Light Switch Plate_v1 (Autodesk Fusion 360 design; units mm, degrees)
Autodesk Fusion 360 part; units mm, degrees
note: some values were not read from the file. Set by a fixed rule: which sketch regions a step uses.
sketch "Sketch1" plane through (0, 0, 0) normal (0, 0, 1) x (1, 0, 0)
  line L0 (-35, 57) -> (35, 57)
  line L1 (35, 57) -> (35, -57)
  line L2 (35, -57) -> (-35, -57)
  line L3 (-35, -57) -> (-35, 57)
  line L4 (-50, 0) -> (50, 0)
  circle A0 centre (0.0006, 30.16) radius 3.5
  circle A1 centre (0.0006, -30.16) radius 3.5
  line L5 (0, 65) -> (0, -65)
  line L6 (5.155, 0) -> (5.155, 11.965)
  line L7 (5.155, 11.965) -> (0, 11.965)
  line L8 (-5.155, 11.965) -> (0, 11.965)
  line L9 (-5.155, 0) -> (-5.155, 11.965)
  line L10 (-5.155, 0) -> (-5.155, -11.965)
  line L11 (5.155, -11.965) -> (0, -11.965)
  line L12 (5.155, 0) -> (5.155, -11.965)
  line L13 (-5.155, -11.965) -> (0, -11.965)
  circle A2 centre (0.0006, 30.16) radius 2.25
  circle A3 centre (0.0006, -30.16) radius 2.25
  circle A4 centre (0.0006, 30.16) radius 5
  circle A5 centre (0.0006, -30.16) radius 5
  circle A6 centre (21, 45) radius 2.5
  circle A7 centre (-21, 45) radius 2.5
  circle A8 centre (21, -45) radius 2.5
  circle A9 centre (-21, -45) radius 2.5
  circle A10 centre (16, 0) radius 2.5
  circle A11 centre (-16, 0) radius 2.5
  line L14 (31, 53) -> (-31, 53)
  line L15 (-31, 53) -> (-31, -53)
  line L16 (-31, -53) -> (31, -53)
  line L17 (31, -53) -> (31, 53)
  dimension "d1" = 60.32
  dimension "d3" = 10.31
  dimension "d4" = 23.93
  dimension "d5" = 4.5
  dimension "d6" = 10
  dimension "d7" = 5
  dimension "d8" = 114
  dimension "d9" = 5
  dimension "d24" = 7
  constraint horizontal L0
  constraint vertical L1
  constraint horizontal L2
  constraint vertical L3
  constraint perpendicular L1 L4
  constraint symmetric L4 A0 A1
  constraint perpendicular L4 L5
  constraint coincident L4 L6.start
  constraint perpendicular L4 L6
  constraint coincident L5 L7.end
  constraint perpendicular L5 L7
  constraint symmetric L5 L6.start L9.start
  constraint symmetric L5 L6.end L8.start
  constraint symmetric L5 L7.end L8.end
  constraint symmetric L4 L6.start L12.start
  constraint symmetric L4 L6.end L11.start
  constraint symmetric L4 L7.end L11.end
  constraint symmetric L4 L8.start L10.end
  constraint symmetric L4 L9.start L10.start
  constraint concentric A0 A2
  constraint symmetric L4 A2 A3
  constraint concentric A0 A4
  constraint symmetric L4 A4 A5
  constraint symmetric L5 A6 A7
  constraint symmetric L4 A6 A8
  constraint symmetric L4 A7 A9
  constraint coincident L4 A10.centre
  constraint symmetric L5 A10 A11
  constraint horizontal L14
  constraint vertical L15
  constraint horizontal L16
  constraint vertical L17
  measures "d1" distance of A0.centre A1.centre
  measures "d3" distance of L10.end L11.start
  measures "d4" distance of L6.end L11.start
  measures "d5" diameter of A2
  measures "d6" diameter of A4
  measures "d7" diameter of A6
  measures "d8" distance of L0.end L1.end
  measures "d9" diameter of A10
  measures "d24" diameter of A0
extrude "Extrude1" add sketch "Sketch1" along normal blind 5.5 contours L0 L3 L4 L5 L14 L15 | L0 L1 L4 L5 L14 L17 | L2 L3 L4 L5 L15 L16 | L1 L2 L4 L5 L16 L17 makes body 1
extrude "Extrude2" add sketch "Sketch1" along normal blind 3 separate body contours L4 A11 | L4 A11 | L4 A10 | L4 A10 | A6 | A7 | A8 | A9 makes body 2 at (23.4969, -45.1246, 2) makes body 3 at (-13.5124, -0.2489, 1) makes body 4 at (-18.5031, 44.8754, 2) makes body 5 at (-18.5031, -45.1246, 2) makes body 6 at (18.4876, -0.2489, 1) makes body 7 at (23.4969, 44.8754, 2)
extrude "Extrude3" add sketch "Sketch1" along normal blind 2 contours L4 L5 L6 L7 A4 A10 L14 L17 | L4 L5 L8 L9 A4 A11 L14 L15 | L4 L5 L10 L13 A5 A11 L15 L16 | L4 L5 L11 L12 A5 A10 L16 L17 bodies 1 2 3 4 5 6 7
chamfer "Chamfer1" distance 2.5 distance2 3.5 4 edges at (-31, 0, 5.5) (0, 53, 5.5) (31, 0, 5.5) (0, -53, 5.5) measured on face at (33.6667, -17.6667, 5.5) measured on face at (33.6667, -17.6667, 5.5) measured on face at (33.6667, -17.6667, 5.5) measured on face at (33.6667, -17.6667, 5.5) on bodies 1
chamfer "Chamfer2" distance 2 distance2 3.5 4 edges at (35, 0, 0) (0, -57, 0) (-35, 0, 0) (0, 57, 0) measured on face at (-25.0517, 3.9883, 0) measured on face at (-25.0517, 3.9883, 0) measured on face at (-25.0517, 3.9883, 0) measured on face at (-25.0517, 3.9883, 0) on bodies 1
extrude "Extrude4" add sketch "Sketch1" along normal blind 4 contours A0 L5 A4 | A0 L5 A4 | A0 L5 A2 | A0 L5 A2 | A1 L5 A5 | A1 L5 A5 | A1 L5 A3 | A1 L5 A3 bodies 1
chamfer "Chamfer3" distance 2.5 distance2 1.25 2 edges at (-2.0971, -29.3464, 0) (-2.0971, 30.9736, 0) measured on face at (2.2394, -29.936, 1.3333) measured on face at (2.2394, 30.384, 1.3333) on bodies 1
